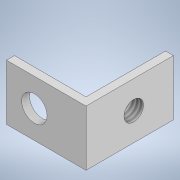
# Autodesk Inventor part: Single Thrd Right Support Farnell1466883
Saved by Autodesk Inventor 2021 (Build 250183000, 183)
## iProperties
Created: 2020-08-04
Part Number: Single Thrd Right Support Farnell1466883
Material: Generic
Document SubType Name: Modeling
Designer: jgray
Density: 1 g/cm^3
Appearance: Default
Author: jgray
Autodesk Inventor part; units mm, degrees
ref_plane "YZ Plane" through (0, 0, 0) normal (1, 0, 0) x (0, 1, 0)
ref_plane "XZ Plane" through (0, 0, 0) normal (0, 1, 0) x (-1, 0, 0)
ref_plane "XY Plane" through (0, 0, 0) normal (0, 0, 1) x (1, 0, 0)
sketch "Sketch1" plane through (0, 0, 0) normal (0, 1, 0) x (-1, 0, 0)
  line L0 (1, -11) -> (0, -11)
  line L1 (0, -11) -> (0, 0)
  line L2 (0, 0) -> (10, 0)
  line L3 (10, 0) -> (10, -1)
  line L4 (9, -1) -> (1, -1)
  line L5 (1, -1) -> (1, -10)
  line L6 (1, -10) -> (1, -11)
  line L7 (9, -1) -> (10, -1)
  dimension "d0" = 10
  dimension "d1" = 11
  dimension "d2" = 1
  constraints: 16 end point, 3 perpendicular, 2 parallel, 1 coincident, 1 horizontal, 1 other
  measures "d0" distance of L1.end L2.end
  measures "d1" distance of L0.end L1.end
  measures "d2" distance between parallel lines of L2 L4
extrude "Extrusion1" add sketch "Sketch1" along normal blind 7
sketch "Sketch2" plane through (-10, 0, 0) normal (0, 0, 1) x (1, 0, 0)
  line L0 (-7.7219, 3.5) -> (14.6275, 3.5)
  line L1 (3.5, 11.0535) -> (3.5, -3.5767)
  line L2 (10, 0) -> (10, 7) projected
  line L3 (0, 0) -> (0, 7) projected
  point P0 (10, 3.5)
  point P1 (3.5, 3.5)
  dimension "d13" = 6.5
  constraints: 4 end point, 3 point on line, 1 horizontal, 1 midpoint, 1 vertical
  measures "d13" distance between parallel lines of L2 L1
hole "Hole1" at (-6.5, 3.5, 0) direction (0, 0, -1) diameter 3.2 end through all clearance for "Flat Head Machine Screw" size "M3" standard "Ansi Metric M Profile"
sketch "Sketch3" plane through (-1, 0, -11) normal (-1, 0, 0) x (0, 0, 1)
  line L0 (5, -6.7291) -> (5, 15.8224)
  line L1 (-2.4783, 3.5) -> (17.6078, 3.5)
  line L2 (0, 0) -> (10, 0) projected
  line L3 (10, 0) -> (10, 7) projected
  line L4 (0, 7) -> (10, 7) projected
  line L5 (0, 0) -> (0, 7) projected
  line L6 (11, 0) -> (11, 7) projected
  circle A0 centre (5, 3.5) radius 2
  point P0 (0, 3.5)
  dimension "d14" = 6
  dimension "d15" = 4
  constraints: 4 end point, 3 point on line, 1 centre point, 1 horizontal, 1 midpoint, 1 vertical
  measures "d14" distance between parallel lines of L0 L6
  measures "d15" diameter of A0
extrude "Extrusion2" add sketch "Sketch3" along normal blind 1 contours A0 L1 L0 | L0 L1 A0 | L1 A0 L0 | L0 A0 L1
fillet "Fillet1" radius 0.4 1 edges at (-1, 3.5, -8)
sketch "Sketch4" plane through (-2, 3.5, -6) normal (-1, 0, 0) x (0, 0, 1)
  point P0 (6, -3.5)
  point P1 (0, 0)
hole "Hole2" at (-2, 3.5, -6) direction (1, 0, 0) diameter 2.459 end through all thread size "M3x0.5" class "6H" standard "ISO Metric profile"
body "Solid1"
